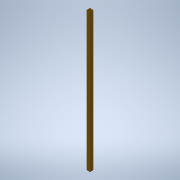
# Autodesk Inventor part: metalon2
Saved by Autodesk Inventor 2020 (Build 240168000, 168)
## iProperties
Created: 2016-02-19
Part Number: metalon2
Material: Genérico
Document SubType Name: Modeling
Designer: al131100X
Density: 1 g/cm^3
Appearance: Padrão
Author: al131100X
Autodesk Inventor part; units mm, degrees
ref_plane "YZ Plane" through (0, 0, 0) normal (1, 0, 0) x (0, 1, 0)
ref_plane "XZ Plane" through (0, 0, 0) normal (0, 1, 0) x (-1, 0, 0)
ref_plane "XY Plane" through (0, 0, 0) normal (0, 0, 1) x (1, 0, 0)
sketch "Sketch1" plane through (0, 0, 0) normal (0, 1, 0) x (-1, 0, 0)
  line L0 (18.2419, 23.2079) -> (57.2419, 23.2079)
  line L1 (57.7419, 22.7079) -> (57.7419, -16.2921)
  line L2 (57.2419, -16.7921) -> (18.2419, -16.7921)
  line L3 (17.7419, -16.2921) -> (17.7419, 22.7079)
  line L4 (56.2419, 21.7079) -> (19.2419, 21.7079)
  line L5 (19.2419, 21.7079) -> (19.2419, -15.2921)
  line L6 (19.2419, -15.2921) -> (56.2419, -15.2921)
  line L7 (56.2419, -15.2921) -> (56.2419, 21.7079)
  arc A0 (18.2419, 23.2079) -> (17.7419, 22.7079) centre (18.2419, 22.7079) ccw
  arc A1 (57.7419, 22.7079) -> (57.2419, 23.2079) centre (57.2419, 22.7079) ccw
  arc A2 (57.2419, -16.7921) -> (57.7419, -16.2921) centre (57.2419, -16.2921) ccw
  arc A3 (17.7419, -16.2921) -> (18.2419, -16.7921) centre (18.2419, -16.2921) ccw
  point P0 (0, 0)
  point P1 (17.7419, 23.2079)
  point P2 (57.7419, 23.2079)
  point P3 (57.7419, -16.7921)
  dimension "d0" = 40
  dimension "d1" = 40
  dimension "d2" = 1.5
  dimension "d3" = 0.5
  constraints: 16 end point, 8 point on circle, 8 tangent, 6 point on line, 4 centre point, 4 perpendicular, 3 equal radius, 2 parallel, 1 horizontal, 3 other
  measures "d0" distance of point (17.742, 23.208) point (57.742, 23.208)
  measures "d1" distance of point (57.742, 23.208) point (57.742, -16.792)
  measures "d2" distance between parallel lines of L0 L4
  measures "d3" radius of A0
extrude "Extrusion1" add sketch "Sketch1" along normal blind 1635
body "Solid1"
